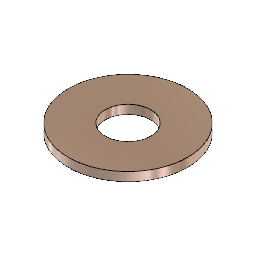
SHVFeedthroughFilterWithPulseLine (Autodesk Fusion 360 archive; units mm, degrees)
design "Washer"
Autodesk Fusion 360 part; units mm, degrees
note: some values were not read from the file. Set by a fixed rule: the direction of a hole.
sketch "Sketch1" plane through (0, 0, 0) normal (0, 0, 1) x (1, 0, 0)
  circle A0 centre (0, 0) radius 8.5
  circle A1 centre (0, 0) radius 3.2385
  dimension "d1" = 17
  dimension "d2" = 6.477
  constraint coincident A0.centre A1.centre
  measures "d1" diameter of A0
  measures "d2" diameter of A1
extrude "Extrude1" add sketch "Sketch1" along normal blind 1.27
sketch "Sketch2" plane through (0, 0, 0) normal (0, 0, -1) x (1, 0, 0)
  arc A0 (-2.7777, 8.0333) -> (2.7777, 8.0333) centre (0, 15) ccw
  circle A1 centre (0, 0) radius 8.5
  line L0 (0, -1.75) -> (0, -22.5)
  dimension "d6" = 15
  dimension "d10" = 7.5
  constraint coincident A0.end A1
  constraint coincident A0.start A1
  constraint coincident A0.centre L0
  measures "d6" distance of A1.centre A0.centre
  measures "d10" radius of A0
extrude "Extrude2" [rolled back] taper angle 0
pattern_circular "C-Pattern1" [rolled back] total angle 360

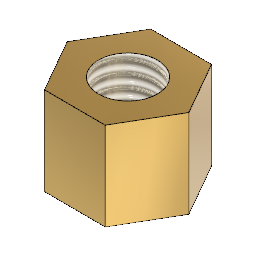
design "CapacitorArrayCenter"
Autodesk Fusion 360 part; units mm, degrees
sketch "Sketch1" plane through (0, 0, 0) normal (0, 0, 1) x (1, 0, 0)
  line L0 (1.7454, 2.9923) -> (-1.7187, 3.0077)
  line L1 (-1.7187, 3.0077) -> (-3.4641, 0.0154)
  line L2 (-3.4641, 0.0154) -> (-1.7454, -2.9923)
  line L3 (-1.7454, -2.9923) -> (1.7187, -3.0077)
  line L4 (1.7187, -3.0077) -> (3.4641, -0.0154)
  line L5 (3.4641, -0.0154) -> (1.7454, 2.9923)
  dimension "d1" = 6
  measures "d1" distance of L0 L3
extrude "Extrude1" add sketch "Sketch1" along normal mid plane 5
sketch "Sketch2" plane through (0, 0, 2.5) normal (0, 0, 1) x (-1, 0, 0)
  line L0 (-3.4641, 0.0154) -> (-1.7454, -2.9923)
  line L1 (-1.7454, -2.9923) -> (1.7187, -3.0077)
  line L2 (1.7187, -3.0077) -> (3.4641, -0.0154)
  line L3 (3.4641, -0.0154) -> (1.7454, 2.9923)
  line L4 (1.7454, 2.9923) -> (-1.7187, 3.0077)
  line L5 (-1.7187, 3.0077) -> (-3.4641, 0.0154)
hole "Hole1" at (0, 0, 2.5) direction (0, 0, -1) diameter 3.332 end through all
thread "Thread1" "ISO Metric profile 4.0 M4x0.7 6H" major diameter 4.1095 minor diameter 3.332 pitch 0.7 angle 60 resizes the face on face at (0.083, -1.6639, 0.8333)

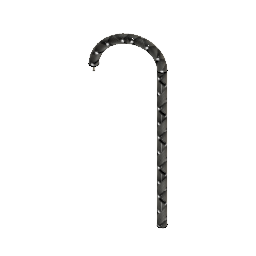
design "LMR-100"
Autodesk Fusion 360 part; units mm, degrees
sketch "Sketch2" plane through (0, 0, 0) normal (0, 0, 1) x (-1, 0, 0)
  circle A0 centre (-10.92, 0) radius 1.055
  line L0 (-10.92, 0) -> (0, 7.8)
  line L1 (-5.46, 3.9) -> (-2.6743, 0)
  dimension "d28" = 2.11
  dimension "d29" = 7.8
  dimension "d31" = 10.92
  constraint coincident A0.centre L0.start
  constraint midpoint L0 L1.start
  constraint perpendicular L0 L1
  constraint vertical origin L0.end
  constraint horizontal origin A0.centre
  constraint horizontal origin L1.end
  measures "d28" diameter of A0
  measures "d29" distance of origin L0.end
  measures "d31" distance of origin A0.centre
revolve "Revolve1" add sketch "Sketch2" angle 180 about axis through (5.46, -3.9, 0) along (0.581238, -0.813733, 0) makes body 1
sketch "Sketch3" plane through (0, 0, 0) normal (0, 0, -1) x (1, 0, 0)
  circle A0 centre (10.92, 0) radius 1.055
extrude "Extrude2" add sketch "Sketch3" along normal blind 36.8 bodies 1
sketch "Sketch6" plane through (0, 0, 0) normal (0, 0, -1) x (1, 0, 0)
  circle A0 centre (0, 7.8) radius 0.25
  circle A1 centre (0, 7.8) radius 1.055
  dimension "d25" = 0.5
  constraint coincident A0.centre A1.centre
  measures "d25" diameter of A0
extrude "Extrude3" add sketch "Sketch6" along normal blind 1.6 separate body contours A0 makes body 2
equation "d7 = 50 mm - 13.2 mm"
equation "d31 = ( 0.75 in + 2.79 mm ) / 2"
equation "d17 = 74 mm - 10.8 mm"

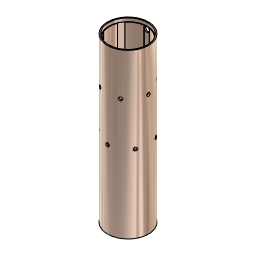
design "OuterTube"
Autodesk Fusion 360 part; units mm, degrees
sketch "Sketch1" plane through (0, 0, 0) normal (0, 0, 1) x (1, 0, 0)
  circle A0 centre (0, 0) radius 9.525
  circle A1 centre (0, 0) radius 8.7122
  dimension "d1" = 19.05
  dimension "d2" = 0.8128
  constraint coincident A0.centre A1.centre
  constraint concentric A0 A1
  measures "d1" diameter of A0
  measures "d2" distance of A0 A1
extrude "Extrude1" add sketch "Sketch1" along normal blind 76
sketch "Sketch2" plane through (0, 0, 0) normal (1, 0, 0) x (0, 1, 0)
  line L0 (0, 1.75) -> (0, 22.5)
  point P0 (0, 8)
  dimension "d8" = 8
  constraint coincident P0 L0
  measures "d8" distance of origin P0
hole "Hole1" at (0, 0, 8) direction (-1, 0, 0) diameter 2.3813 depth 30 tip angle 118
sketch "Sketch3" plane through (0, 0, 0) normal (0, 1, 0) x (1, 0, 0)
  point P0 (0, -36)
  dimension "d9" = 36
  measures "d9" distance of origin P0
hole "Hole2" at (0, 0, 36) direction (0, -1, 0) diameter 1.5875 depth 20 tip angle 118
pattern_circular "C-Pattern1" count 6 over 360 about axis through (0, 0, 1.75) along (0, 0, 1) of "Hole2"
sketch "Sketch4" plane through (0, 0, 0) normal (0, 0, -1) x (1, 0, 0)
  circle A0 centre (0, 0) radius 8.7122
  circle A1 centre (0, 0) radius 9.525
  circle A2 centre (0, 0) radius 9
  dimension "d15" = 18
  constraint coincident A0.centre A1.centre
  measures "d15" diameter of A2
extrude "Extrude2" cut sketch "Sketch4" against normal blind 1.5 contours A2
sketch "Sketch5" plane through (0, 0, 76) normal (0, 0, 1) x (-1, 0, 0)
  circle A0 centre (0, 0) radius 8.7122
  circle A1 centre (0, 0) radius 9.525
  circle A2 centre (0, 0) radius 9
  dimension "d18" = 18
  constraint concentric A0 A2
  measures "d18" diameter of A2
extrude "Extrude3" cut sketch "Sketch5" against normal blind 1.5 contours A2
sketch "Sketch6" plane through (0, 0, 0) normal (0, 1, 0) x (1, 0, 0)
  line L0 (-9.525, -76) -> (9.525, -76)
  point P0 (0, -73.2094)
  dimension "d21" = 2.7906
  measures "d21" distance of P0 L0
hole "Hole3" at (0, 0, 73.2094) direction (0, 1, 0) diameter 2.3813 end through all
sketch "Sketch7" plane through (0, 0, 0) normal (1, 0, 0) x (0, 1, 0)
  line L0 (9.525, 0) -> (-9.525, 0)
  point P0 (0, 56.25)
  dimension "d25" = 56.25
  measures "d25" distance of P0 L0
hole "Hole4" at (0, 0, 56.25) direction (-1, 0, 0) diameter 1.5875 end through all
pattern_circular "C-Pattern2" count 6 over 360 about axis through (0, 0, 1.75) along (0, 0, 1) of "Hole4"
sketch "Sketch8" plane through (0, 0, 0) normal (0, 0, -1) x (1, 0, 0)
  circle A0 centre (0, 0) radius 9
  circle A1 centre (0, 0) radius 9.525
  line L0 (7.064, 5.5449) -> (8.334, 3.3451)
  line L1 (8.334, 3.3451) -> (-7.064, -5.5449)
  line L2 (-7.064, -5.5449) -> (-8.334, -3.3451)
  line L3 (-8.334, -3.3451) -> (7.064, 5.5449)
  line L4 (1.75, 0) -> (22.5, 0)
  line L5 (0, -1.75) -> (0, -22.5)
  line L6 (-0.635, 1.0999) -> (0, 0)
  line L7 (0, 0) -> (7.699, 4.445)
  point P0 (-0.635, 1.0999)
  point P1 (7.699, 4.445)
  dimension "d31" = 17.78
  dimension "d32" = 2.54
  dimension "d38" = 30
  constraint coincident A0.centre A1.centre
  constraint perpendicular L0 L3
  constraint perpendicular L1 L2
  constraint parallel L1 L3
  constraint midpoint L3 P0
  constraint midpoint L0 P1
  constraint coincident P0 L6.start
  constraint coincident P1 L7.end
  constraint perpendicular L3 L6
  constraint perpendicular L0 L7
  measures "d31" distance of L0.start L2.end
  measures "d32" distance of L0.start L0.end
  measures "d38" angle of L1 L4
extrude "Extrude4" cut sketch "Sketch8" against normal through all contours L0 L3 L6 L7 | L0 L1 L2 L3 L6 L7
pattern_circular "C-Pattern3" count 3 over 360 about axis through (0, 0, 1.75) along (0, 0, 1) of "Extrude4"
equation "d6 = 3 in / 32"
equation "d11 = 1 in / 16"
equation "d21 = 1.6 mm + 3 in / 64"
equation "d23 = 3 in / 32"
equation "d27 = 1 in / 16"

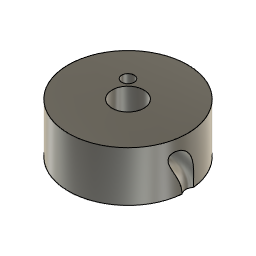
design "EndCap"
Autodesk Fusion 360 part; units mm, degrees
sketch "Sketch1" plane through (0, 0, 0) normal (0, 0, 1) x (1, 0, 0)
  circle A0 centre (0, 0) radius 9.525
  circle A1 centre (0, -7.8) radius 1.4
  circle A2 centre (10.925, 0) radius 1.4
  line L0 (1.75, 0) -> (22.5, 0)
  circle A3 centre (0.6608, 2.301) radius 11.919
  line L1 (0, -7.8) -> (0.6608, 2.301)
  line L2 (0.6608, 2.301) -> (10.925, 0)
  line L3 (-0.6294, 4.025) -> (15.7848, 0.3453)
  line L4 (-1.6049, -10.8865) -> (-0.6294, 4.025)
  line L5 (0.6608, 2.301) -> (7.8023, -7.2416)
  dimension "d1" = 19.05
  dimension "d30" = 7.8
  dimension "d31" = 2.8
  dimension "d32" = 81.107
  constraint coincident A0.centre origin
  constraint vertical A0.centre A1.centre
  constraint equal A1 A2
  constraint tangent A0 A2
  constraint coincident A2.centre L0
  constraint tangent A2 A3
  constraint tangent A0 A3
  constraint coincident A1.centre L1.start
  constraint coincident A3.centre L1.end
  constraint coincident A2.centre L2.end
  constraint parallel L2 L3
  constraint tangent A2 L3
  constraint parallel L1 L4
  constraint tangent A1 L4
  constraint coincident L3.start L4.end
  constraint coincident A3 L5.end
  measures "d1" diameter of A0
  measures "d30" vertical distance of A0.centre A1.centre
  measures "d31" diameter of A1
  measures "d32" angle of L1 L2
extrude "Extrude1" add sketch "Sketch1" along normal blind 8
ref_plane "WorkPlane3" through (8.4015, -6.7623, 3.0831) normal (0.649448, -0.760406, 0) x (-0.760406, -0.649448, 0)
sketch "Sketch8" plane through (8.4015, -6.7623, 3.0831) normal (0.649448, -0.760406, 0) x (-0.760406, -0.649448, 0)
  arc A0 (-9.401, 3.0831) -> (10.87, 3.0831) centre (0.7345, 3.0831) ccw
  arc A1 (-6.068, 3.0831) -> (7.537, 3.0831) centre (0.7345, 3.0831) ccw
  line L0 (10.87, 3.0831) -> (7.537, 3.0831)
  line L1 (-6.068, 3.0831) -> (-9.401, 3.0831)
  line L2 (-11.919, 3.0831) -> (11.919, 3.0831)
  dimension "d34" = 3.333
  dimension "d39" = 7.537
  dimension "d40" = 6.068
  constraint horizontal L0
  constraint parallel L0 L1
  constraint equal L0 L1
  constraint coincident A0.centre L0
  constraint coincident A0.centre L1
  constraint coincident A0.centre A1.centre
  constraint coincident A0.centre L2
  measures "d34" distance of A0.end A1.end
  measures "d39" horizontal distance of origin A1.end
  measures "d40" horizontal distance of origin A1.start
emboss "Emboss2" [suppressed]
fillet "Fillet3" [suppressed]
extrude "Extrude4" cut sketch "Sketch1" along normal through all of body 1 contours A0 L0 L2 L5 | A0 L0 L5 | A0 A1 L1 L2 L3 L4 | A0 A1 L1 L4 L5 | A0 L3 L4 | A1 keep common part
sketch "Sketch9" plane through (0, 0, 0) normal (0, 0, 1) x (1, 0, 0)
hole "Hole3" at (0, 0, 0) direction (0, 0, 1) diameter 5.08 end through all countersink diameter 10 countersink angle 60
sketch "Sketch10" plane through (0, 0, 8) normal (0, 0, 1) x (-1, 0, 0)
  circle A0 centre (0, 0) radius 2.54
  circle A1 centre (0, 0) radius 9.525
  circle A2 centre (2.8284, -2.8284) radius 1
  line L0 (2.8284, -2.8284) -> (0, 0)
  line L1 (0, -1.75) -> (0, -22.5)
  circle A3 centre (0, 0) radius 5
  dimension "d49" = 2
  dimension "d50" = 45
  constraint coincident A2.centre L0.start
  constraint coincident A0.centre A1.centre
  constraint tangent A2 A3
  measures "d49" diameter of A2
  measures "d50" angle of L0 L1
extrude "Extrude5" cut sketch "Sketch10" against normal through all contours A2
sketch "Sketch11" plane through (0, 0, 0) normal (0, 0, -1) x (1, 0, 0)
  circle A0 centre (0, 0) radius 5
  circle A1 centre (0, 0) radius 8.725
  circle A2 centre (0, 0) radius 9.525
  dimension "d52" = 0.8
  constraint coincident A0.centre A1.centre
  measures "d52" distance of A1 A2
extrude "Extrude6" cut sketch "Sketch11" against normal blind 0.5 contours A0 | A1
revolve "Revolve1" cut sketch "Sketch1" angle 180 about axis through (0.6608, 2.301, 0) along (-0.599176, 0.800617, 0) contours A1

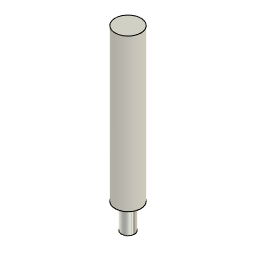
design "LEGENDCable"
Autodesk Fusion 360 part; units mm, degrees
sketch "Sketch1" plane through (0, 0, 0) normal (0, 0, 1) x (1, 0, 0)
  circle A0 centre (0, 0) radius 1.27
  dimension "d1" = 2.54
  constraint coincident A0.centre origin
  measures "d1" diameter of A0
extrude "Extrude1" add sketch "Sketch1" along normal blind 5 makes body 1
sketch "Sketch2" plane through (0, 0, 5) normal (0, 0, 1) x (-1, 0, 0)
  circle A0 centre (0, 0) radius 1.27
  circle A1 centre (0, 0) radius 2.54
  dimension "d4" = 5.08
  constraint coincident A0.centre A1.centre
  measures "d4" diameter of A1
extrude "Extrude2" add sketch "Sketch2" along normal blind 30 separate body contours A0 | A1 makes body 2

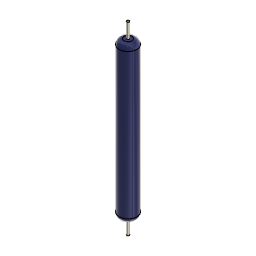
design "MOX1125-22"
Autodesk Fusion 360 part; units mm, degrees
sketch "Sketch1" plane through (0, 0, 0) normal (0, 0, 1) x (1, 0, 0)
  circle A0 centre (0, 0) radius 1.78
  dimension "d1" = 3.56
  constraint coincident A0.centre origin
  measures "d1" diameter of A0
extrude "Extrude1" add sketch "Sketch1" along normal mid plane 31 makes body 1
sketch "Sketch2" plane through (0, 0, 15.5) normal (0, 0, 1) x (-1, 0, 0)
  circle A0 centre (0, 0) radius 1.78
  circle A1 centre (0, 0) radius 0.254
  dimension "d4" = 0.508
  constraint concentric A0 A1
  measures "d4" diameter of A1
extrude "Extrude2" add sketch "Sketch2" along normal blind 3 separate body contours A1 makes body 2
mirror "Mirror1" about plane through (0, 0, 0) normal (0, 0, 1) of "Extrude2" makes body 3
fillet "Fillet1" radius 1 2 edges at (-1.6595, -0.6437, 15.5) (-1.6595, 0.6437, -15.5) on bodies 1

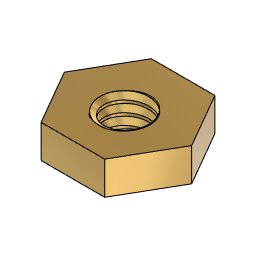
design "M2Nut"
Autodesk Fusion 360 part; units mm, degrees
sketch "Sketch1" plane through (0, 0, 0) normal (0, 0, 1) x (1, 0, 0)
  line L0 (-1.1547, 2) -> (-2.3094, 0)
  line L1 (-2.3094, 0) -> (-1.1547, -2)
  line L2 (-1.1547, -2) -> (1.1547, -2)
  line L3 (1.1547, -2) -> (2.3094, 0)
  line L4 (2.3094, 0) -> (1.1547, 2)
  line L5 (1.1547, 2) -> (-1.1547, 2)
  dimension "d1" = 4
  measures "d1" distance of L2 L5
extrude "Extrude1" add sketch "Sketch1" along normal blind 1.2
sketch "Sketch2" plane through (0, 0, 1.2) normal (0, 0, 1) x (-1, 0, 0)
  line L0 (-1.1547, -2) -> (1.1547, -2)
  line L1 (1.1547, -2) -> (2.3094, 0)
  line L2 (2.3094, 0) -> (1.1547, 2)
  line L3 (1.1547, 2) -> (-1.1547, 2)
  line L4 (-1.1547, 2) -> (-2.3094, 0)
  line L5 (-2.3094, 0) -> (-1.1547, -2)
hole "Hole1" at (0, 0, 1.2) direction (0, 0, -1) diameter 1.623 end through all
thread "Thread1" "ISO Metric profile 2.0 M2x0.4 6H" major diameter 2.074 minor diameter 1.623 pitch 0.4 angle 60 modelled right hand crest width 0.1065 on face at (0.0808, -0.8075, 0.8) crest through (0.8115, 0, 1.1)
